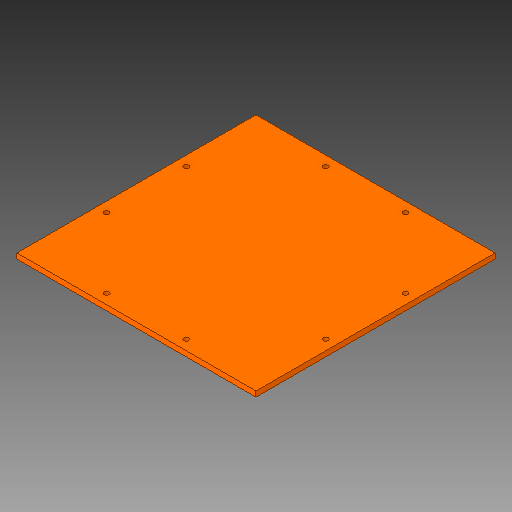
# Autodesk Inventor part: ControlPlate
Saved by Autodesk Inventor 2019 (Build 230136000, 136)
## iProperties
Created: 2019-01-04
Part Number: ControlPlate
Material: Generic
Document SubType Name: Modeling
Designer: james
Density: 1 g/cm^3
Appearance: Default(1)
Author: james
Autodesk Inventor part; units mm, degrees
ref_plane "YZ Plane" through (0, 0, 0) normal (1, 0, 0) x (0, 1, 0)
ref_plane "XZ Plane" through (0, 0, 0) normal (0, 1, 0) x (-1, 0, 0)
ref_plane "XY Plane" through (0, 0, 0) normal (0, 0, 1) x (1, 0, 0)
sketch "Sketch1" plane through (0, 0, 0) normal (0, 1, 0) x (-1, 0, 0)
  line L0 (148.429, 108.1825) -> (-80.171, 108.1825)
  line L1 (-80.171, 108.1825) -> (-80.171, -120.4175)
  line L2 (-80.171, -120.4175) -> (148.429, -120.4175)
  line L3 (148.429, -120.4175) -> (148.429, 108.1825)
  point P0 (0, 0)
  dimension "d0" = 228.6
  dimension "d1" = 228.6
  constraints: 8 end point, 2 parallel, 1 horizontal, 1 perpendicular
  measures "d0" distance of L0.end L1.end
  measures "d1" distance of L0.start L0.end
extrude "Extrusion1" add sketch "Sketch1" along normal blind 5.08
sketch "Sketch2" plane through (0, 5.08, 0) normal (0, 1, 0) x (1, 0, 0)
  line L0 (-148.429, -108.1825) -> (80.171, -108.1825) projected
  line L1 (80.171, 120.4175) -> (-148.429, 120.4175) projected
  line L2 (-148.429, 120.4175) -> (-148.429, -108.1825) projected
  line L3 (80.171, -108.1825) -> (80.171, 120.4175) projected
  point P0 (0, 0)
  point P1 (-138.904, -31.9825)
  point P2 (-138.904, 44.2175)
  point P3 (-72.229, 110.8925)
  point P4 (3.971, 110.8925)
  point P5 (70.646, 44.2175)
  point P6 (70.646, -31.9825)
  point P7 (-72.229, -98.6575)
  point P8 (3.971, -98.6575)
  dimension "d4" = 76.2
  dimension "d5" = 76.2
  dimension "d6" = 76.2
  dimension "d7" = 9.525
  dimension "d8" = 9.525
  dimension "d9" = 76.2
  dimension "d10" = 9.525
  dimension "d11" = 76.2
  dimension "d12" = 9.525
  dimension "d13" = 9.525
  measures "d4" distance from line of L0 point (-138.904, -31.983)
  measures "d5" distance of point (-138.904, 44.217) point (-138.904, -31.983)
  measures "d6" distance from line of L1 point (-138.904, 44.217)
  measures "d7" distance from line of L2 point (-138.904, 44.217)
  measures "d8" distance from line of L2 point (-138.904, -31.983)
  measures "d9" distance from line of point (-72.229, 110.892) L2
  measures "d10" distance from line of L1 point (-72.229, 110.892)
  measures "d11" distance of point (3.971, 110.892) point (-72.229, 110.892)
  measures "d12" distance from line of L3 point (70.646, 44.217)
  measures "d13" distance from line of L0 point (-72.229, -98.658)
hole "Hole1" at (-138.904, 5.08, 31.9825) at (-138.904, 5.08, -44.2175) at (-72.229, 5.08, -110.8925) at (3.971, 5.08, -110.8925) at (70.646, 5.08, -44.2175) at (70.646, 5.08, 31.9825) at (-72.229, 5.08, 98.6575) at (3.971, 5.08, 98.6575) direction (0, -1, 0) diameter 4.826 end through all
equation "\"d0\" = ControlPlateLength"
equation "\"d1\" = ControlPlateLength"
equation "\"d2\" = WallWidth"
equation "\"d7\" = ControlHoleBoltHoleMid"
equation "\"d8\" = ControlHoleBoltHoleMid"
equation "\"d10\" = ControlHoleBoltHoleMid"
equation "\"d12\" = ControlHoleBoltHoleMid"
equation "\"d13\" = ControlHoleBoltHoleMid"
equation "\"DSLength\" = 1371.6"
equation "\"DSWidth\" = 304.8"
equation "\"DCDeckHeight\" = 76.2"
equation "\"WallWidth\" = 5.08"
equation "\"EdgeAngle\" = 10deg"
equation "\"LengthCuts\" = 152.4"
equation "\"WidthCuts\" = 50.8"
equation "\"PartLength\" = 228.6"
equation "\"PartWidth\" = 152.4"
equation "\"BoltHoldDiam\" = 6.35"
equation "\"ControlPlateLength\" = 228.6"
equation "\"ControlPlateWidth\" = 228.6"
equation "\"ControlPlateShelfLength\" = 19.05"
equation "\"ControlHoleLength\" = 190.5"
equation "\"ControlHoleWidth\" = 190.5"
equation "\"ControlHoleFromSide\" = 63.5"
equation "\"ControlHoleBoltHoleMid\" = 9.525"
equation "\"DU1CHLength\" = 146.05"
equation "\"DU1CHWidth\" = 69.85"
equation "\"CPFromBack\" = 63.5"
equation "\"CPDeckHeight\" = 71.12"
equation "\"CPFromSide\" = 63.5"
equation "\"ControlPlateScrewLength\" = 76.2"
equation "\"DSBackHeight\" = 127"
equation "\"BackShelf\" = 25.4"
equation "\"MainAngle\" = 168.22deg"
equation "\"CPDWidthHole\" = 120.65"
equation "\"CPDLengthHole\" = 146.05"
equation "\"DownBackHeight\" = 130.7084"
body "Solid1"
